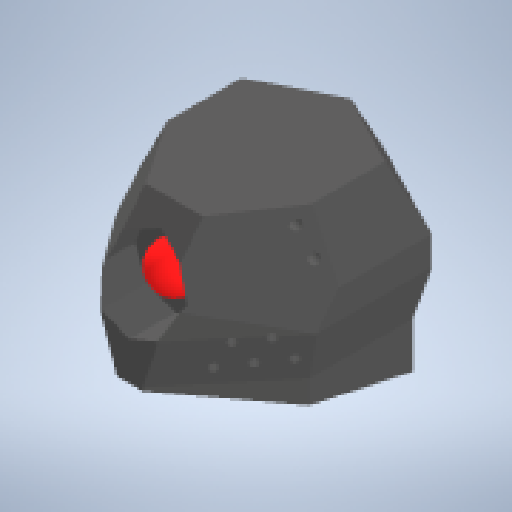
# Autodesk Inventor part: head_bace
Saved by Autodesk Inventor 2024.1 (Build 281209000, 209)
## iProperties
Created: 2024-02-25
Part Number: head_bace
Material: 一般
Document SubType Name: Modeling
Designer: hibik
Density: 1 g/cm^3
Appearance: 既定
Author: hibik
Autodesk Inventor part; units mm, degrees
ref_plane "YZ Plane" through (0, 0, 0) normal (1, 0, 0) x (0, 1, 0)
ref_plane "XZ Plane" through (0, 0, 0) normal (0, 1, 0) x (-1, 0, 0)
sketch "スケッチ1" plane through (0, 0, 0) normal (0, 1, 0) x (-1, 0, 0)
  line L0 (-17.5, -21) -> (0, 0)
  line L1 (0, 0) -> (17.5, -21)
  line L2 (17.5, -21) -> (17.5, -41)
  line L3 (17.5, -41) -> (0, -50)
  line L4 (0, -50) -> (-17.5, -41)
  line L5 (-17.5, -41) -> (-17.5, -21)
  line L6 (0, -60) -> (0, 10) projected
  line L7 (24.5, 0) -> (-24.5, 0) projected
  dimension "d0" = 50
  dimension "d12" = 35
  dimension "d13" = 20
  dimension "d14" = 21
  constraints: 12 end point, 2 horizontal alignment, 1 coincident, 1 point on line, 1 vertical, 2 other
  measures "d0" distance of L0.end L3.end
  measures "d12" distance between parallel lines of L5 L2
  measures "d13" distance of L4.end L0.start
  measures "d14" vertical distance of L0.end L1.end
extrude "押し出し1" add sketch "スケッチ1" along normal blind 18
chamfer "面取り1" distance 5 distance2 10 6 edges at (8.75, 18, -10.5) (17.5, 18, -31) (8.75, 18, -45.5) (-8.75, 18, -45.5) (-17.5, 18, -31) (-8.75, 18, -10.5) measured on face at (8.3659, 18, -10.8201) measured on face at (-8.3659, 18, -10.8201) measured on face at (8.5213, 18, -45.0554) measured on face at (17, 18, -31) measured on face at (-17, 18, -31) measured on face at (-8.5213, 18, -45.0554)
extrude "押し出し2" add sketch "スケッチ1" against normal blind 5
ref_plane "作業平面1" through (0, 8, 0) normal (0, -0.7881104, 0.6155339) x (1, 0, 0)
sketch "スケッチ2" plane through (0, 8, 0) normal (0, -0.7881104, 0.6155339) x (1, 0, 0)
  line L0 (0, 0) -> (17.5, -16.5503) projected
  line L1 (-17.5, -16.5503) -> (0, 0) projected
  line L2 (-5, -4.7287) -> (-5, -4.7287)
  line L3 (-5, -4.7287) -> (5, -4.7287)
  line L4 (13.3346, -12.611) -> (5, -4.7287)
  line L5 (-5, -4.7287) -> (-23.6413, -26.9446)
  line L6 (5, -4.7287) -> (18.7173, -21.0763)
  line L7 (-23.6413, -26.9446) -> (-26.2109, -24.7885)
  line L8 (-26.2109, -24.7885) -> (-17.5, -16.5503)
  line L9 (17.5, -16.5503) -> (23.8178, -21.8516)
  line L10 (23.8178, -21.8516) -> (18.7173, -21.0763)
  point P0 (0, -4.9243)
  dimension "d9" = 10
  dimension "d25" = 130
  dimension "d26" = 130
  constraints: 18 end point, 4 point on line, 2 collinear, 1 horizontal, 1 parallel
  measures "d9" distance of L2.end L3.end
  measures "d25" angle of L3 L5
  measures "d26" angle of L6 L3
extrude "押し出し3" cut sketch "スケッチ2" against normal through all
chamfer "面取り2" distance 2 distance2 8 6 edges at (-8.75, -5, -10.5) (-17.5, -5, -31) (-8.75, -5, -45.5) (8.75, -5, -45.5) (17.5, -5, -31) (8.75, -5, -10.5) measured on face at (17, -5, -31) measured on face at (-8.5213, -5, -45.0554) measured on face at (8.3659, -5, -10.8201) measured on face at (-17, -5, -31) measured on face at (-8.3659, -5, -10.8201) measured on face at (8.5213, -5, -45.0554)
sketch "スケッチ3" plane through (0, -5, 0) normal (0, -1, 0) x (1, 0, 0)
  line L0 (0, -3.1241) -> (15.5, -21.7241) projected
  line L1 (-15.5, -21.7241) -> (0, -3.1241) projected
  line L2 (-15.5, -39.7796) -> (-15.5, -21.7241) projected
  line L3 (0, -47.751) -> (-15.5, -39.7796) projected
  line L4 (15.5, -39.7796) -> (0, -47.751) projected
  line L5 (15.5, -21.7241) -> (15.5, -39.7796) projected
  point P0 (0, 0)
extrude "押し出し4" add sketch "スケッチ3" along normal blind 8
ref_plane "作業平面2" through (0, -5, -3.1241) normal (0, -0.9770022, 0.2132292) x (-0.3818297, -0.1970734, -0.9029774)
sketch "スケッチ4" plane through (0, -5, -3.1241) normal (0, -0.9770022, 0.2132292) x (-0.3818297, -0.1970734, -0.9029774)
  line L0 (80, -28.4848) -> (-10, -28.4848)
  line L1 (-10, -28.4848) -> (-10, 40)
  line L2 (-10, 40) -> (80, 40)
  line L3 (80, 40) -> (80, -28.4848)
  point P0 (-3.8064, -1.5725)
  constraints: 8 end point, 2 parallel, 1 horizontal, 1 perpendicular
extrude "押し出し5" cut sketch "スケッチ4" along normal through all
ref_plane "作業平面3" through (-5, 8, -6) normal (0, 0, 1) x (1, 0, 0)
sketch "スケッチ5" plane through (-5, 8, -6) normal (0, 0, 1) x (1, 0, 0)
  line L0 (-30, 20) -> (40, 20)
  line L1 (40, 20) -> (40, -30)
  line L2 (40, -30) -> (-30, -30)
  line L3 (-30, -30) -> (-30, 20)
  point P0 (5, -8)
  constraints: 8 end point, 2 parallel, 1 horizontal, 1 perpendicular
extrude "押し出し6" cut sketch "スケッチ5" along normal through all
sketch "スケッチ6" plane through (-5, 8, -6) normal (0, 0, 1) x (1, 0, 0)
  line L0 (0, 0) -> (10, 0) projected
  circle A0 centre (5, 0) radius 5
  line L1 (9.9497, -4.9497) -> (5, -7)
  line L2 (5, -7) -> (0.0503, -4.9497)
  line L3 (0.0503, -4.9497) -> (-2, 0)
  line L4 (-2, 0) -> (0.0503, 4.9497)
  line L5 (0.0503, 4.9497) -> (5, 7)
  line L6 (5, 7) -> (9.9497, 4.9497)
  line L7 (9.9497, 4.9497) -> (12, 0)
  line L8 (12, 0) -> (9.9497, -4.9497)
  point P0 (5, -8)
  dimension "d29" = 7
  constraints: 16 end point, 2 midpoint, 1 coincident, 1 horizontal alignment, 1 vertical alignment, 19 other
  measures "d29" distance of point (5, 0) L5.end
extrude "押し出し7" cut sketch "スケッチ6" against normal blind 8 contours A0 L0 | L0 A0 | L1 L2 L3 L4 L5 L6 L7 L8
sketch "スケッチ8" plane through (-5, 8, -14) normal (0, 0, 1) x (1, 0, 0)
  line L0 (5, 0) -> (-12.5, 0) projected
  circle A0 centre (5, 0) radius 4
  line L1 (5, 4) -> (5, -4)
  line L2 (5, -5) -> (5, 0) projected
  point P0 (5, -8)
  dimension "d32" = 8
  constraints: 2 end point, 2 point on circle, 1 centre point, 1 midpoint, 1 point on line
  measures "d32" diameter of A0
revolve "回転1" add sketch "スケッチ8" angle 360 about axis through (0, 12, -14) along (0, -1, 0) contours L1 A0
sketch "スケッチ9" plane through (-15.5, -5, -21.7241) normal (-0.7452841, -0.2425356, 0.6210701) x (0.6214323, 0.0848617, 0.7788584)
  circle A0 centre (10.2962, 6.6564) radius 0.8
  circle A1 centre (12.0048, 1.9574) radius 0.8
  circle A2 centre (7.081, 2.8272) radius 0.8
  circle A3 centre (2.1573, 3.697) radius 0.8
  circle A4 centre (5.3724, 7.5262) radius 0.8
  line L0 (2.1573, 3.697) -> (7.081, 2.8272) construction
  line L1 (7.081, 2.8272) -> (12.0048, 1.9574) construction
  line L2 (12.0048, 1.9574) -> (7.081, 2.8272)
  line L3 (5.3724, 7.5262) -> (10.2962, 6.6564) construction
  line L4 (10.2962, 6.6564) -> (9.5429, 2.3923) construction
  line L5 (5.3724, 7.5262) -> (4.6191, 3.2621) construction
  line L6 (10.2962, 6.6564) -> (12.0048, 1.9574) construction
  line L7 (12.0048, 1.9574) -> (11.7379, 0.4469) construction
  line L8 (12.0048, 1.9574) -> (13.2927, 2.4257) construction
  line L9 (20.3897, -1.7904) -> (19.4508, 6.57) projected
  line L10 (0, 0) -> (20.3897, -1.7904) projected
  point P0 (26.9765, 2.9875)
  dimension "d34" = 1.6
  dimension "d35" = 5
  dimension "d36" = 5
  dimension "d37" = 7.9143
  dimension "d38" = 3
  constraints: 18 end point, 5 centre point, 4 equal radius, 4 perpendicular, 3 equal length, 2 midpoint, 1 collinear
  measures "d34" diameter of A1
  measures "d35" distance from line of L0.end L7
  measures "d36" distance from line of L3.end L8
  measures "d37" distance from line of L9 L1.end
  measures "d38" distance from line of L10 L1.end
extrude "押し出し8" cut sketch "スケッチ9" against normal blind 5
sketch "スケッチ10" plane through (-12.5, 18, -25.1515) normal (-0.7660444, 0.3956576, 0.5065876) x (0.5515991, 0, 0.8341093)
  circle A0 centre (2.1738, -2.388) radius 0.8 projected
  circle A1 centre (0.2082, -6.8935) radius 0.8 projected
  point P0 (27.8741, -17.8951)
extrude "押し出し9" cut sketch "スケッチ10" against normal blind 5
mirror "ミラー1" about plane through (0, 0, 0) normal (1, 0, 0) of "押し出し8", "押し出し9"
sketch "スケッチ11" plane through (0, -5, -3.1241) normal (0, -0.9770022, 0.2132292) x (0.9242327, -0.0814172, -0.3730484)
  line L0 (3.339, -1.8055) -> (-1.091, -3.6357) projected
  line L1 (-7.0564, -23.5137) -> (-1.091, -3.6357) projected
  line L2 (0, -40.594) -> (-7.0564, -23.5137) projected
  line L3 (28.6512, -28.7573) -> (0, -40.594) projected
  line L4 (21.5948, -11.677) -> (28.6512, -28.7573) projected
  line L5 (3.339, -1.8055) -> (21.5948, -11.677) projected
  line L6 (0, -40.594) -> (21.5948, -11.677)
  line L7 (-7.0564, -23.5137) -> (28.6512, -28.7573)
  circle A0 centre (10.7974, -26.1355) radius 4.25
  point P0 (-1.5725, 3.8064)
  dimension "d43" = 8.5
  constraints: 4 end point, 1 centre point, 1 midpoint
  measures "d43" diameter of A0
extrude "押し出し10" cut sketch "スケッチ11" against normal blind 1 contours A0 L7 L6 | L6 L7 A0 | L7 L6 A0 | A0 L6 L7
sketch "スケッチ12" plane through (0, -10.0527, -30.9651) normal (0, -0.9770022, 0.2132292) x (1, 0, 0)
  circle A0 centre (0, 0) radius 4.25 projected
  circle A1 centre (0, 0) radius 0.8
  point P0 (0, 32.3965)
  dimension "d46" = 1.6
  constraints: 1 centre point, 1 coincident
  measures "d46" diameter of A1
extrude "押し出し11" cut sketch "スケッチ12" against normal blind 5 contours A1
